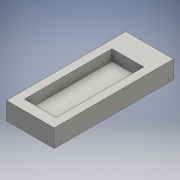
# Autodesk Inventor part: Prueba1MPU
Saved by Autodesk Inventor 2016 (Build 200138000, 138)
## iProperties
Created: 2016-04-24
Part Number: Prueba1MPU
Material: Generic
Document SubType Name: Modeling
Designer: Freddy Chang
Density: 1 g/cm^3
Appearance: Default
Author: Freddy Chang
Autodesk Inventor part; units mm, degrees
ref_plane "YZ Plane" through (0, 0, 0) normal (1, 0, 0) x (0, 1, 0)
ref_plane "XZ Plane" through (0, 0, 0) normal (0, 1, 0) x (-1, 0, 0)
ref_plane "XY Plane" through (0, 0, 0) normal (0, 0, 1) x (1, 0, 0)
sketch "Sketch1" plane through (0, 0, 0) normal (0, 0, 1) x (1, 0, 0)
  line L0 (0, 0) -> (24, 0)
  line L1 (24, 0) -> (24, -60)
  line L2 (24, -60) -> (0, -60)
  line L3 (0, -60) -> (0, 0)
  dimension "d0" = 24
  dimension "d1" = 60
  constraints: 8 end point, 2 parallel, 1 horizontal, 1 perpendicular
  measures "d0" distance of L1.end L2.end
  measures "d1" distance of L0.end L1.end
extrude "Extrusion1" add sketch "Sketch1" along normal blind 9
sketch "Sketch2" plane through (0, 0, 9) normal (0, 0, 1) x (1, 0, 0)
  line L0 (0, -60) -> (24, -60) projected
  line L1 (4, -55) -> (4, -10.95)
  line L2 (20, -10.95) -> (20, -55)
  line L3 (4, -10.95) -> (20, -10.95)
  line L4 (4, -55) -> (20, -55)
  line L5 (24, -60) -> (24, 0) projected
  line L6 (0, 0) -> (0, -60) projected
  line L7 (24, 0) -> (0, 0) projected
  dimension "d7" = 4
  dimension "d8" = 4
  dimension "d9" = 5
  dimension "d10" = 10.95
  constraints: 8 end point, 2 horizontal, 1 parallel
  measures "d7" distance between parallel lines of L5 L2
  measures "d8" distance between parallel lines of L6 L1
  measures "d9" distance between parallel lines of L0 L4
  measures "d10" distance between parallel lines of L7 L3
extrude "Extrusion2" cut sketch "Sketch2" against normal blind 5.5 contours L1 L3 L2 L4
sketch "Sketch3" plane through (24, -60, 0) normal (1, 0, 0) x (0, 0, -1)
  circle A0 centre (-1.5, 3) radius 0.5
  circle A1 centre (-1.5, 57) radius 0.5
  line L0 (0, 0) -> (-9, 0) projected
  line L1 (-9, 0) -> (-9, 60) projected
  line L2 (0, 60) -> (-9, 60) projected
  dimension "d15" = 1
  dimension "d18" = 1
  dimension "d19" = 3
  dimension "d20" = 7.5
  dimension "d21" = 3
  dimension "d22" = 7.5
  constraints: 2 centre point
  measures "d15" diameter of A0
  measures "d18" diameter of A1
  measures "d19" distance from line of L0 A0.centre
  measures "d20" distance from line of L1 A0.centre
  measures "d21" distance from line of L2 A1.centre
  measures "d22" distance from line of L1 A1.centre
extrude "Extrusion3" cut sketch "Sketch3" against normal blind 24
body "Solid1"
